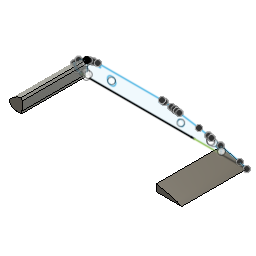
Wing rib packing tape v2 - front & back shapes for 3d printing (Autodesk Fusion 360 design; units mm, degrees)
Autodesk Fusion 360 part; units mm, degrees
sketch "Sketch1" plane through (0, 0, 0) normal (0, 0, 1) x (1, 0, 0) in component "Airfoil structure"
  spline S0 degree 5 poles (152.7645, 9.7049) (152.9716, 9.6615) (153.4494, 9.5595) (154.3565, 9.3601) (155.9477, 9.0023) (158.563, 8.408) (161.765, 7.6797) (165.4684, 6.8398) (169.5125, 5.9246) (173.6689, 4.9817) (177.6907, 4.06) (181.3486, 3.2014) (184.473, 2.4316) (186.9959, 1.7512) (188.9984, 1.125) (190.7574, 0.4718) (192.2494, -0.1494) (193.5536, -0.7078) (194.5245, -1.1262) (195.0353, -1.3469) knots 0 0 0 0 0 0 0.066667 0.133333 0.2 0.266667 0.333333 0.4 0.466667 0.533333 0.6 0.666667 0.733333 0.8 0.866667 0.933333 1 1 1 1 1 1
  line L0 (151.6776, 9.9322) -> (153.8514, 9.4775)
  line L1 (191.9867, -0.0294) -> (198.0838, -2.6644)
  circle A0 centre (33.1388, 9.1296) radius 4.765
  circle A1 centre (116.1615, 7.0362) radius 3.175
  spline S1 degree 5 poles (-3.078, -1.3469) (-3.5988, -1.2541) (-4.5389, -1.0768) (-5.6443, -0.8357) (-6.5925, -0.5673) (-7.3281, -0.2956) (-8.0506, 0.0085) (-9.0186, 0.5701) (-10.0677, 1.7864) (-10.9637, 3.2509) (-11.5101, 4.486) (-11.5777, 5.0948) (-11.4072, 5.6425) (-11.0115, 6.6062) (-10.1312, 7.9923) (-8.6029, 9.6425) (-6.4042, 11.2716) (-4.197, 12.5713) (-2.7351, 13.406) (-1.8317, 13.8945) (-1.0217, 14.2663) (0.0954, 14.6934) (1.4589, 15.1916) (2.6392, 15.6172) (3.2971, 15.8534) knots 0 0 0 0 0 0 0.05 0.1 0.15 0.2 0.25 0.3 0.35 0.4 0.45 0.5 0.55 0.6 0.65 0.7 0.75 0.8 0.85 0.9 0.95 1 1 1 1 1 1
  line L2 (0.5733, -1.9976) -> (-6.7293, -0.6962)
  line L3 (-0.0118, 14.6656) -> (6.606, 17.0412)
  line L4 (-8.4792, 9.8153) -> (-3.9569, 12.8132)
  line L5 (-11.5034, 4.2257) -> (-11.5345, 5.6935)
  line L6 (-7.2174, -0.5359) -> (-9.7443, 1.1286)
  line L7 (19.5688, 19.3646) -> (90.5688, 19.3646)
  spline S2 degree 5 poles (93.5688, 19.3646) (93.8188, 19.3387) (94.2829, 19.2905) (94.8714, 19.229) (95.4658, 19.1659) (96.0263, 19.1049) (96.567, 19.0445) (97.2368, 18.9678) (98.1315, 18.8622) (99.313, 18.7173) (100.8214, 18.5245) (102.3118, 18.3263) (103.5973, 18.1504) (104.53, 18.0207) (105.0153, 17.9528) knots 0 0 0 0 0 0 0.1 0.2 0.3 0.4 0.5 0.6 0.7 0.8 0.9 1 1 1 1 1 1
  line L8 (92.266, 19.4996) -> (94.8715, 19.2297)
  line L9 (103.6448, 18.1447) -> (106.3858, 17.761)
  spline S3 degree 5 poles (6.5765, 16.943) (6.9079, 17.0449) (7.5374, 17.2364) (8.3817, 17.4868) (9.3156, 17.7508) (10.2084, 17.9865) (10.8922, 18.156) (11.4504, 18.29) (11.9864, 18.4184) (12.6265, 18.5675) (13.504, 18.76) (14.4962, 18.9637) (15.447, 19.1503) (16.1786, 19.2906) (16.5688, 19.3646) knots 0 0 0 0 0 0 0.1 0.2 0.3 0.4 0.5 0.6 0.7 0.8 0.9 1 1 1 1 1 1
  line L10 (5.4107, 16.5846) -> (7.7424, 17.3015)
  line L11 (15.2328, 19.111) -> (17.9048, 19.6183)
  line L12 (152.2841, 9.8053) -> (152.7645, 9.7049)
  line L13 (107.9851, 17.5282) -> (108.4359, 17.4637)
  line L14 (6.1441, 16.7993) -> (6.5765, 16.943)
  line L15 (128.8618, -1.3469) -> (132.3168, -1.3469)
  line L16 (149.3476, 10.4194) -> (148.7335, 7.483)
  line L17 (148.7335, 7.483) -> (151.67, 6.8689)
  line L18 (151.67, 6.8689) -> (152.2841, 9.8053)
  line L19 (3.2971, 15.8534) -> (4.243, 13.0064)
  line L20 (4.243, 13.0064) -> (7.09, 13.9524)
  line L21 (7.09, 13.9524) -> (6.1441, 16.7993)
  line L22 (161.1951, -1.3469) -> (161.1951, 1.6531)
  line L23 (161.1951, 1.6531) -> (164.1951, 1.6531)
  line L24 (164.1951, 1.6531) -> (164.1951, -1.3469)
  line L25 (132.3168, -1.3469) -> (161.1951, -1.3469)
  line L26 (164.1951, -1.3469) -> (195.0353, -1.3469)
  line L27 (3.4543, -1.3469) -> (3.4543, 1.6531)
  line L28 (3.4543, 1.6531) -> (6.4543, 1.6531)
  line L29 (6.4543, 1.6531) -> (6.4543, -1.3469)
  line L30 (-3.078, -1.3469) -> (3.4543, -1.3469)
  line L31 (6.4543, -1.3469) -> (128.8618, -1.3469)
  line L32 (105.0153, 17.9528) -> (107.9851, 17.5282)
  line L33 (19.5688, 19.3646) -> (19.5688, 16.3646)
  line L34 (19.5688, 16.3646) -> (16.5688, 16.3646)
  line L35 (16.5688, 16.3646) -> (16.5688, 19.3646)
  line L36 (90.5688, 19.3646) -> (90.5688, 16.3646)
  line L37 (90.5688, 16.3646) -> (93.5688, 16.3646)
  line L38 (93.5688, 16.3646) -> (93.5688, 19.3646)
  line L39 (113.7881, 13.5683) -> (110.8279, 14.0557)
  line L40 (110.8279, 14.0557) -> (111.3153, 17.0159)
  line L41 (113.7881, 13.5683) -> (114.2755, 16.5285)
  spline S4 degree 5 poles (108.4359, 17.4637) (108.5255, 17.4506) (108.6943, 17.4261) (108.916, 17.394) (109.1532, 17.3597) (109.3785, 17.3272) (109.5651, 17.2997) (109.7467, 17.2719) (109.9518, 17.2393) (110.199, 17.1992) (110.5008, 17.1497) (110.7926, 17.1018) (111.0419, 17.0608) (111.2219, 17.0312) (111.3153, 17.0159) knots 0 0 0 0 0 0 0.1 0.2 0.3 0.4 0.5 0.6 0.7 0.8 0.9 1 1 1 1 1 1
  line L42 (107.9387, 17.5361) -> (108.933, 17.3913)
  line L43 (110.8712, 17.0888) -> (111.7595, 16.9429)
  spline S5 degree 5 poles (114.2755, 16.5285) (114.908, 16.4243) (116.2157, 16.2103) (118.305, 15.8728) (121.3361, 15.3892) (125.4662, 14.728) (129.833, 14.0131) (134.2929, 13.2559) (138.6571, 12.4806) (142.6792, 11.7322) (146.0525, 11.0804) (147.9853, 10.6961) (148.8914, 10.5134) (149.2384, 10.4423) (149.3476, 10.4194) knots 0 0 0 0 0 0 0.1 0.2 0.3 0.4 0.5 0.6 0.7 0.8 0.9 1 1 1 1 1 1
  line L44 (111.4536, 16.9935) -> (117.0973, 16.0636)
  line L45 (148.6356, 10.5684) -> (150.0597, 10.2705)
  line L46 (151.67, 6.8689) -> (155.718, 6.0223) construction
  line L47 (164.1951, 1.6531) -> (164.6963, 1.6531) construction
  line L48 (152.6756, 9.7234) -> (152.0615, 6.787)
  line L49 (164.1951, 1.6531) -> (164.9867, 2.4447) construction
  line L50 (164.1951, 1.6531) -> (164.8816, 1.6531) construction
  line L51 (164.5909, 2.0489) -> (164.5909, -1.3469)
  line L52 (152.2841, 9.8053) -> (152.6756, 9.7234) construction
  line L53 (152.6756, 9.7234) -> (151.9827, 6.4137) construction
  line L54 (151.5912, 6.4957) -> (152.2841, 9.8053) construction
  line L55 (152.2841, 9.8053) -> (152.6756, 9.7234)
  line L56 (152.6756, 9.7234) -> (151.9342, 6.1818)
  line L57 (151.9342, 6.1818) -> (151.5427, 6.2638) construction
  line L58 (151.5427, 6.2638) -> (152.2841, 9.8053)
  line L59 (2.9567, -1.3469) -> (2.9567, 2.1507)
  line L60 (2.9567, 2.1507) -> (3.8737, 2.1507)
  line L61 (3.8737, 2.1507) -> (3.8737, 12.5773)
  line L62 (3.8737, 12.5773) -> (2.8398, 15.6891)
  line L63 (4.243, 13.0064) -> (1.9707, 12.2515) construction
  line L64 (3.4543, 1.6531) -> (2.143, 2.9644) construction
  line L65 (3.4543, 1.6531) -> (5.3087, 1.6531) construction
  line L66 (164.5909, 2.0489) -> (152.0615, 6.787)
  line L67 (151.67, 6.8689) -> (152.3309, 5.404) construction
  line L68 (151.5764, 6.4249) -> (164.1951, 1.6531)
  line L69 (164.5909, 2.0489) -> (164.5909, 7.0392)
  point P0 (-8.4808, 0.2964)
  point P1 (-11.5189, 4.9596)
  point P2 (-6.2181, 11.3142)
  point P3 (11.4183, 18.2822)
  point P4 (96.5722, 19.0435)
  point P5 (109.7229, 17.2753)
  point P6 (137.8507, 12.6179)
  point P7 (163.7235, 7.2358)
  point P8 (186.7896, 1.7868)
  dimension "d38" = 77
  dimension "d53" = 9.53
  dimension "d54" = 6.35
  dimension "d59" = 3
  dimension "d65" = 0.4
  dimension "d68" = 3
  dimension "d69" = 3
  dimension "d73" = 45
  dimension "d81" = 135
  dimension "d82" = 3
  dimension "d83" = 3
  dimension "d88" = 45
  constraint midpoint S0.start L0
  constraint midpoint S0.end L1
  constraint midpoint S1.start L2
  constraint midpoint S1.end L3
  constraint midpoint P2 L4
  constraint midpoint P1 L5
  constraint midpoint P0 L6
  constraint horizontal L7
  constraint midpoint S2.start L8
  constraint midpoint S2.end L9
  constraint midpoint S3.start L10
  constraint midpoint S3.end L11
  constraint parallel L25 L30
  constraint collinear L25 L30
  constraint horizontal L30
  constraint parallel L15 L25
  constraint perpendicular L12 L16
  constraint perpendicular L16 L17
  constraint perpendicular L12 L18
  constraint perpendicular L14 L19
  constraint perpendicular L19 L20
  constraint perpendicular L14 L21
  constraint perpendicular L22 L25
  constraint perpendicular L22 L23
  constraint perpendicular L23 L24
  constraint collinear L25 L26
  constraint perpendicular L27 L30
  constraint perpendicular L27 L28
  constraint coincident L29.end L30
  constraint perpendicular L29 L30
  constraint collinear L30 L31
  constraint vertical L33
  constraint horizontal L34
  constraint vertical L35
  constraint vertical L36
  constraint horizontal L37
  constraint vertical L38
  constraint equal L36 L38
  constraint equal L36 L37
  constraint perpendicular L39 L40
  constraint perpendicular L39 L41
  constraint midpoint L13.end L42
  constraint midpoint L40.end L43
  constraint midpoint L41.end L44
  constraint midpoint L16.start L45
  constraint perpendicular L18 L46
  constraint perpendicular L24 L47
  constraint coincident S0 L48.start
  constraint coincident L46 L48.end
  constraint perpendicular L46 L48
  constraint equal L17 L18
  constraint equal L16 L17
  constraint equal L22 L23
  constraint perpendicular L18 L45
  constraint perpendicular L0 L18
  constraint horizontal L50
  constraint midpoint L49 L51.start
  constraint coincident L26 L51.end
  constraint parallel L24 L51
  constraint perpendicular L52 L53
  constraint parallel L53 L54
  constraint perpendicular L55 L56
  constraint parallel L55 L57
  constraint parallel L56 L58
  constraint coincident S1 L62.end
  constraint parallel L27 L59
  constraint parallel L19 L62
  constraint perpendicular L19 L63
  constraint vertical L61
  constraint horizontal L65
  constraint coincident L59.end L64
  constraint equal L27 L28
  constraint equal L19 L20
  constraint parallel L60 L65
  constraint coincident L54 L68.start
  constraint parallel L66 L68
  constraint coincident S0 L69.end
  constraint parallel L51 L69
  measures "d38" distance of S3.end S2.start
  measures "d53" diameter of A0
  measures "d54" diameter of A1
  measures "d59" distance of L36.end L37.end
  measures "d65" distance of L18 L48
  measures "d68" distance of L16.end L17.end
  measures "d69" distance of L22.end L23.end
  measures "d73" angle of L49 L50
  measures "d81" angle of L64 L65
  measures "d82" distance of L19.end L20.end
  measures "d83" distance of L27.end L28.end
  measures "d88" angle of L66 L67
extrude "Extrude4" add sketch "Sketch1" along normal blind 77.78 contours S1 L30 L59 L60 L61 L62 makes body 1 in component "Airfoil structure"
extrude "Extrude3" add sketch "Sketch1" along normal blind 77.78 separate body contours S0 L26 L51 L69 makes body 2
extrude "Extrude3'" [suppressed] in component "Airfoil structure"
sketch "Sketch3" plane through (0, 0, 0) normal (0, 0, 1) x (1, 0, 0)
component "Airfoil structure" placed x (1, 0, 0) y (0, 1, 0) z (0, 0, 1) at (0, 0, 0)
named bodies: "FrontShape", "BackShape"
